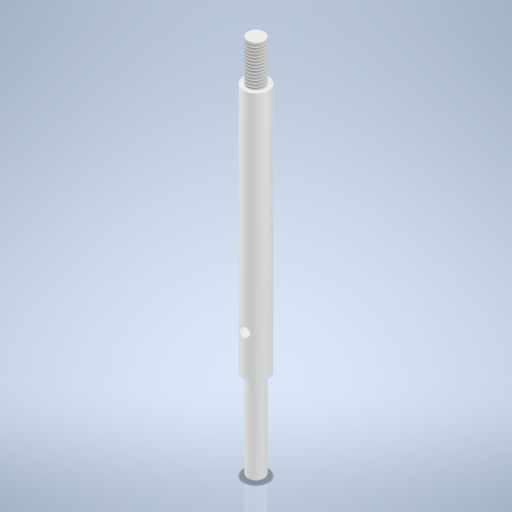
# Autodesk Inventor part: 205 part 1
Saved by Autodesk Inventor 2024 (Build 280153000, 153)
## iProperties
Created: 2024-07-12
Part Number: 205 part 1
Material: Aluminium 6061
Document SubType Name: Modeling
Designer: ffogue
Density: 2.7 g/cm^3
Appearance: Aluminium - flach
Author: ffogue
Autodesk Inventor part; units mm, degrees
ref_plane "YZ Plane" through (0, 0, 0) normal (1, 0, 0) x (0, 1, 0)
ref_plane "XY Plane" through (0, 0, 0) normal (0, 0, 1) x (1, 0, 0)
sketch "Skizze1" plane through (0, 0, 0) normal (0, 1, 0) x (-1, 0, 0)
  line L0 (0, 0) -> (2, 0)
  line L1 (2, 0) -> (2, -10)
  line L2 (2, -10) -> (3, -10)
  line L3 (3, -10) -> (3, -71)
  line L4 (3, -71) -> (2, -71)
  line L5 (2, -71) -> (2, -93)
  line L6 (2, -93) -> (0, -93)
  line L7 (0, -93) -> (0, 0)
  dimension "d0" = 10
  dimension "d1" = 22
  dimension "d2" = 93
  dimension "d3" = 4
  dimension "d4" = 6
  constraints: 16 end point, 6 perpendicular, 2 point on line, 1 horizontal
  measures "d0" distance between parallel lines of L2 L0
  measures "d1" distance between parallel lines of L6 L4
  measures "d2" distance between parallel lines of L6 L0
  measures "d3" diameter of L5 L7
  measures "d4" diameter of L3 L7
revolve "Umdrehung1" add sketch "Skizze1" angle 360 about axis through (0, 0, -93) along (0, 0, 1)
thread "Gewinde1" size "M4x0.7" class "6g" standard "ISO Metric profile" full length
ref_plane "Arbeitsebene1" through (0, 3, 0) normal (0, 1, 0) x (-1, 0, 0)
sketch "Skizze2" plane through (0, 3, 0) normal (0, 1, 0) x (-1, 0, 0)
  line L0 (3, -10) -> (-3, -10) projected
  line L1 (3, -71) -> (-3, -71) projected
  point P0 (0, 0)
  point P1 (0, -61)
  dimension "d9" = 10
  constraints: 1 vertical alignment
  measures "d9" distance from line of L1 point (0, -61)
hole "Bohrung1" at (0, 3, -61) direction (0, -1, 0) diameter 2.5 end through all
chamfer "Fasen1" distance 0.5 angle 45 1 edges at (2, 0, -93)
